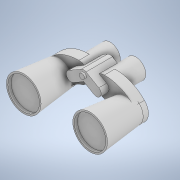
# Autodesk Inventor part: Część19
Saved by Autodesk Inventor 2021 (Build 250183000, 183)
## iProperties
Created: 2023-10-31
Part Number: Część19
Material: Ogólny
Document SubType Name: Modeling
Designer: Jakub
Density: 1 g/cm^3
Appearance: Domyślna
Author: Jakub
Autodesk Inventor part; units mm, degrees
ref_plane "YZ Plane" through (0, 0, 0) normal (1, 0, 0) x (0, 1, 0)
ref_plane "XZ Plane" through (0, 0, 0) normal (0, 1, 0) x (-1, 0, 0)
ref_plane "XY Plane" through (0, 0, 0) normal (0, 0, 1) x (1, 0, 0)
sketch "Szkic1" plane through (0, 0, 0) normal (0, 0, 1) x (1, 0, 0)
  circle A0 centre (0, 0) radius 5
  line L0 (0, 0) -> (-108.8243, -62.8298)
  line L1 (0, 0) -> (125.6595, 0) construction
  line L2 (0, 0) -> (0, -14)
  line L3 (0, -14) -> (-24.2487, -14)
  line L4 (-24.2487, -14) -> (-32.0429, -18.5)
  line L5 (-32.0429, -18.5) -> (-32.0429, -18.5)
  line L6 (-36.5429, -10.7058) -> (-32.0429, -18.5)
  line L7 (0, 0) -> (7.7942, 4.5)
  line L8 (7.7942, 4.5) -> (7.7942, 4.5)
  line L9 (12.2942, -3.2942) -> (7.7942, 4.5)
  line L10 (-4.5, 7.7942) -> (-28.7487, -6.2058)
  line L11 (-19.7487, -21.7942) -> (4.5, -7.7942)
  arc A1 (4.5, -7.7942) -> (7.7942, 4.5) centre (0, 0) ccw
  arc A2 (-32.0429, -18.5) -> (-19.7487, -21.7942) centre (-24.2487, -14) ccw
  arc A3 (-28.7487, -6.2058) -> (-32.0429, -18.5) centre (-24.2487, -14) ccw
  arc A4 (7.7942, 4.5) -> (-4.5, 7.7942) centre (0, 0) ccw
  point P0 (-27.5429, -26.2942)
  point P1 (3.2942, 12.2942)
  dimension "d0" = 10
  dimension "d1" = 150
  dimension "d2" = 14
  dimension "d3" = 9
  dimension "d4" = 9
  dimension "d5" = 18
  dimension "d6" = 9
  dimension "d7" = 9
  dimension "d8" = 18
  dimension "d9" = 9
  constraints: 24 end point, 12 point on line, 8 point on circle, 8 tangent, 5 centre point, 4 perpendicular, 3 equal radius, 1 coincident, 1 equal length, 1 horizontal, 1 vertical
  measures "d0" diameter of A0
  measures "d1" angle of L0 L1
  measures "d2" distance of L0.start L2.end
  measures "d3" distance of L3.end L4.end
  measures "d4" distance of L4.end L6.start
  measures "d5" distance of L6.start point (-27.543, -26.294)
  measures "d6" distance of L0.start L7.end
  measures "d7" distance of L7.end L9.start
  measures "d8" distance of L9.start point (3.294, 12.294)
  measures "d9" radius of A1
extrude "Wyciągnięcie proste1" add sketch "Szkic1" along normal mid plane 50 contours A0 L7 A1 L11 L2 | A0 L0 A3 L10 A4 L7 | L2 L11 L3 L0 A0 | L3 L11 A2 L0
sketch "Szkic2" plane through (0, 0, 0) normal (0, 0, 1) x (1, 0, 0)
  circle A0 centre (0, 0) radius 5
  constraints: 1 centre point, 1 coincident
extrude "Wyciągnięcie proste2" add sketch "Szkic2" along normal mid plane 57
sketch "Szkic3" plane through (0, 0, 0) normal (0, 0, 1) x (1, 0, 0)
  arc A0 (-28.7487, -6.2058) -> (-19.7487, -21.7942) centre (-24.2487, -14) ccw projected
  circle A1 centre (-24.2487, -14) radius 19
  point P0 (0, 0)
  dimension "d14" = 38
  constraints: 1 centre point, 1 coincident
  measures "d14" diameter of A1
extrude "Wyciągnięcie proste3" add sketch "Szkic3" along normal blind 10 and the other way blind 50
sketch "Szkic4" plane through (0, 0, 0) normal (0, 0, 1) x (1, 0, 0)
  arc A0 (-28.7487, -6.2058) -> (-19.7487, -21.7942) centre (-24.2487, -14) ccw projected
  circle A1 centre (-24.2487, -14) radius 19
  circle A2 centre (0, 0) radius 5 projected
  line L0 (0, 0) -> (141.5882, 0) construction
  arc A3 (-14.2573, 2.1608) -> (-5.2573, -13.4276) centre (-24.2487, -14) ccw projected
  line L1 (-24.2487, -14) -> (-63.2199, -36.5)
  circle A4 centre (-63.2199, -36.5) radius 25
  arc A5 (-24.2487, 5) -> (-80.5692, -18.5) centre (-25.6054, -70.9879) ccw
  arc A6 (-19.7487, -32.4594) -> (-40.7032, -47.3628) centre (-9.5006, -69.0514) ccw
  point P0 (-19.7487, -32.4594)
  point P1 (-24.2487, 5)
  dimension "d20" = 45
  dimension "d21" = 50
  dimension "d22" = 76
  dimension "d24" = 38
  constraints: 8 point on circle, 4 centre point, 4 end point, 2 coincident, 1 horizontal
  measures "d20" distance of L1.start L1.end
  measures "d21" diameter of A4
  measures "d22" radius of A5
  measures "d24" radius of A6
extrude "Wyciągnięcie proste4" add sketch "Szkic4" along normal mid plane 20 contours A1 | A6 A4 L1 A1 | L1 A4 A5 A1 | A4
sketch "Szkic5" plane through (0, 0, 0) normal (0, 0, 1) x (1, 0, 0)
  arc A0 (-80.5692, -18.5) -> (-40.7032, -47.3628) centre (-63.2199, -36.5) ccw projected
  circle A1 centre (-63.2199, -36.5) radius 32.99
  point P0 (0, 0)
  dimension "d39" = 65.98
  constraints: 1 centre point, 1 coincident
  measures "d39" diameter of A1
extrude "Wyciągnięcie proste7" add sketch "Szkic5" along normal blind 76 separate body
chamfer "Faza1" distance 76 distance2 7.99 1 edges at (-96.2099, -36.5, 0) measured on face at (-30.3368, -39.1546, 50.6667)
sketch "Szkic7" plane through (-63.2199, -36.5, 76) normal (0, 0, 1) x (1, 0, 0)
  circle A0 centre (0, 0) radius 30
  point P0 (63.2199, 36.5)
  dimension "d45" = 60
  constraints: 1 centre point
  measures "d45" diameter of A0
extrude "Wyciągnięcie proste8" cut sketch "Szkic7" against normal blind 6 bodies 2
sketch "Szkic8" plane through (-24.2487, -14, -50) normal (0, 0, -1) x (-1, 0, 0)
  circle A0 centre (0, 0) radius 16
  point P0 (-24.2487, 14)
  dimension "d48" = 32
  constraints: 1 centre point
  measures "d48" diameter of A0
extrude "Wyciągnięcie proste9" cut sketch "Szkic8" against normal blind 6 bodies 1
mirror "Odbij1" about plane through (0, 0, 0) normal (1, 0, 0) bodies 2 1
